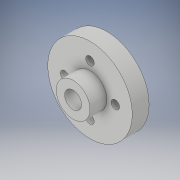
# Autodesk Inventor part: test 2018 1
Saved by Autodesk Inventor 2017 (Build 210142000, 142)
## iProperties
Created: 2018-09-26
Part Number: test 2018 1
Material: Generic
Document SubType Name: Modeling
Designer: qthuynh
Density: 1 g/cm^3
Appearance: Default
Author: qthuynh
Autodesk Inventor part; units mm, degrees
ref_plane "YZ Plane" through (0, 0, 0) normal (1, 0, 0) x (0, 1, 0)
ref_plane "XZ Plane" through (0, 0, 0) normal (0, 1, 0) x (-1, 0, 0)
ref_plane "XY Plane" through (0, 0, 0) normal (0, 0, 1) x (1, 0, 0)
sketch "Sketch1" plane through (0, 0, 0) normal (0, 0, 1) x (1, 0, 0)
  circle A0 centre (0, 0) radius 63.5
  dimension "d0" = 127
  constraints: 1 centre point, 1 coincident
  measures "d0" diameter of A0
extrude "Extrusion1" add sketch "Sketch1" along normal blind 25.4
sketch "Sketch2" plane through (0, 0, 25.4) normal (0, 0, 1) x (1, 0, 0)
  circle A0 centre (0, 0) radius 25.4
  circle A1 centre (0, 0) radius 12.7
  circle A2 centre (0, -38.1) radius 6.35
  circle A3 centre (-38.1, 0) radius 6.35
  dimension "d3" = 50.8
  dimension "d4" = 25.4
  dimension "d5" = 12.7
  dimension "d6" = 38.1
  dimension "d7" = 12.7
  dimension "d8" = 38.1
  constraints: 4 centre point, 2 coincident
  measures "d3" diameter of A0
  measures "d4" diameter of A1
  measures "d5" diameter of A2
  measures "d6" distance of A2.centre A1.centre
  measures "d7" diameter of A3
  measures "d8" distance of A3.centre point (0, 0)
sketch "Sketch3" plane through (0, 0, 25.4) normal (0, 0, 1) x (1, 0, 0)
  circle A0 centre (38.1, 0) radius 6.35
  circle A1 centre (0, 38.1) radius 6.35
  point P0 (0, 0)
  dimension "d9" = 12.7
  dimension "d10" = 38.1
  dimension "d11" = 12.7
  dimension "d12" = 38.1
  constraints: 2 centre point
  measures "d9" diameter of A0
  measures "d10" distance of A0.centre point (0, 0)
  measures "d11" diameter of A1
  measures "d12" distance of point (0, 0) A1.centre
extrude "Extrusion2" add sketch "Sketch2" along normal blind 25.4 contours A0
sketch "Sketch4" plane through (0, 0, 25.4) normal (0, 0, 1) x (1, 0, 0)
  circle A0 centre (-38.1, 0) radius 6.35
  circle A1 centre (0, -38.1) radius 6.35
  point P0 (0, 0)
  dimension "d15" = 12.7
  dimension "d16" = 38.1
  dimension "d17" = 12.7
  dimension "d18" = 38.1
  constraints: 2 centre point
  measures "d15" diameter of A0
  measures "d16" distance of point (0, 0) A0.centre
  measures "d17" diameter of A1
  measures "d18" distance of A1.centre point (0, 0)
extrude "Extrusion3" cut sketch "Sketch3" against normal blind 381 contours A1
extrude "Extrusion4" cut sketch "Sketch4" against normal blind 381
sketch "Sketch5" plane through (0, 0, 25.4) normal (0, 0, 1) x (1, 0, 0)
  circle A0 centre (38.1, 0) radius 6.35
  point P0 (0, 0)
  dimension "d23" = 12.7
  dimension "d24" = 38.1
  constraints: 1 centre point
  measures "d23" diameter of A0
  measures "d24" distance of point (0, 0) A0.centre
extrude "Extrusion5" cut sketch "Sketch5" against normal blind 381
body "Solid1"
